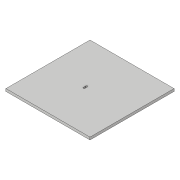
# Autodesk Inventor part: Custom slot
Saved by Autodesk Inventor 2017 (Build 210142000, 142)
## iProperties
Created: 2016-07-23
Part Number: Custom slot
Material: Generic
Document SubType Name: Sheet Metal
Designer: Tutorial Books
Density: 1 g/cm^3
Sheet Metal Rule: Default
Appearance: Default
Author: Tutorial Books
Autodesk Inventor part; units mm, degrees
ref_plane "YZ Plane" through (0, 0, 0) normal (1, 0, 0) x (0, 1, 0)
ref_plane "XZ Plane" through (0, 0, 0) normal (0, 1, 0) x (-1, 0, 0)
ref_plane "XY Plane" through (0, 0, 0) normal (0, 0, 1) x (1, 0, 0)
sketch "Sketch1" plane through (0, 0, 0) normal (0, 1, 0) x (-1, 0, 0)
  line L0 (50.8, 50.8) -> (-50.8, 50.8)
  line L1 (-50.8, 50.8) -> (-50.8, -50.8)
  line L2 (-50.8, -50.8) -> (50.8, -50.8)
  line L3 (50.8, -50.8) -> (50.8, 50.8)
  line L4 (50.8, 50.8) -> (-50.8, -50.8) construction
  line L5 (-50.8, 50.8) -> (50.8, -50.8) construction
  point P0 (0, 0)
  dimension "d0" = 101.6
  dimension "d1" = 101.6
  measures "d0" distance of L2.end L1.end
  measures "d1" distance of L0.end L1.end
extrude "Plate1" add sketch "Sketch1" along normal blind 3.048
sketch "Sketch2" plane through (0, 3.048, 0) normal (0, 1, 0) x (1, 0, 0)
  line L0 (-4.2545, -2.8152) -> (-4.2545, 0.2328) construction
  line L1 (-5.2705, -2.8152) -> (-5.2705, 0.2328)
  line L2 (-3.2385, 0.2328) -> (-3.2385, -2.8152)
  arc A0 (-5.2705, -2.8152) -> (-3.2385, -2.8152) centre (-4.2545, -2.8152) ccw
  arc A1 (-3.2385, 0.2328) -> (-5.2705, 0.2328) centre (-4.2545, 0.2328) ccw
  point P0 (0, 0)
  point P1 (-4.2545, -1.2912)
  point P2 (-4.2545, -1.2912)
  dimension "d3" = 1.016
  dimension "d4" = 3.048
  constraints: 8 end point, 4 point on circle, 4 tangent, 2 centre point, 1 coincident, 1 midpoint, 1 parallel, 1 vertical
  measures "d3" radius of A1
  measures "d4" distance of L0.start L0.end
extrude "Cut1" cut sketch "Sketch2" against normal blind 3.048
equation "\"d3\" = Diameter"
equation "\"d4\" = Length"
equation "\"d5\" = Thickness"
equation "\"BendRadius\" = Thickness"
equation "\"BendReliefWidth\" = Thickness"
equation "\"BendReliefDepth\" = 0.5 * Thickness"
equation "\"CornerReliefSize\" = 4 * Thickness"
equation "\"MinimumRemnant\" = 2 * Thickness"
equation "\"TransitionRadius\" = BendRadius"
equation "\"JacobiRadiusSize\" = BendRadius"
equation "\"GapSize\" = Thickness"
equation "\"d2\" = BendRadius"
equation "\"Diameter\" = 1.016"
equation "\"Length\" = 3.048"
equation "\"Thickness\" = 3.048"
body "Solid1"
